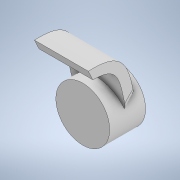
# Autodesk Inventor part: suction_extension
Saved by Autodesk Inventor 2021 (Build 250183000, 183)
## iProperties
Created: 2023-03-20
Part Number: suction_extension
Material: Generic
Document SubType Name: Modeling
Designer: mahmo
Density: 1 g/cm^3
Appearance: Default
Author: mahmo
Autodesk Inventor part; units mm, degrees
ref_plane "YZ Plane" through (0, 0, 0) normal (1, 0, 0) x (0, 1, 0)
ref_plane "XZ Plane" through (0, 0, 0) normal (0, 1, 0) x (-1, 0, 0)
ref_plane "XY Plane" through (0, 0, 0) normal (0, 0, 1) x (1, 0, 0)
sketch "Sketch1" plane through (0, 0, 0) normal (0, 0, 1) x (1, 0, 0)
  circle A0 centre (0, 0) radius 7.5
  dimension "d0" = 15
  constraints: 1 centre point, 1 coincident
  measures "d0" diameter of A0
extrude "Extrusion1" add sketch "Sketch1" along normal blind 10
sketch "Sketch2" plane through (0, 0, 10) normal (0, 0, 1) x (1, 0, 0)
  line L0 (0, 0) -> (0, 15)
  line L1 (-7.5, 16.5) -> (7.5, 16.5)
  line L2 (7.5, 16.5) -> (7.5, 13.5)
  line L3 (7.5, 13.5) -> (-7.5, 13.5)
  line L4 (-7.5, 13.5) -> (-7.5, 16.5)
  line L5 (-7.5, 16.5) -> (7.5, 13.5) construction
  line L6 (7.5, 16.5) -> (-7.5, 13.5) construction
  dimension "d3" = 15
  dimension "d4" = 15
  dimension "d5" = 3
  constraints: 14 end point, 2 midpoint, 2 parallel, 1 horizontal, 1 perpendicular, 1 vertical
  measures "d3" distance of L0.start L0.end
  measures "d4" distance of L2.end L3.end
  measures "d5" distance of L1.end L2.end
sketch "Sketch3" plane through (0, 0, 0) normal (1, 0, 0) x (0, 1, 0)
  line L0 (14.9444, 14.9575) -> (14.9444, 8.9521) construction
  line L1 (14.9444, 8.9521) -> (13.2139, 6.7241) construction
  line L2 (13.2139, 6.7241) -> (8.3998, 6.1566) construction
  line L3 (8.3998, 6.1566) -> (2.9254, 4.977) construction
  spline S0 degree 4 poles (14.9444, 14.9575) (14.9444, 8.9521) (13.2139, 6.7241) (8.3998, 6.1566) (2.9254, 4.977) knots 1 1 1 1 1 2 2 2 2 2
  point P0 (0, 0)
  constraints: 1 vertical, 3 other
sweep "Sweep1" add profiles "Sketch2" path "Sketch3"
fillet "Fillet1" radius 2 2 edges at (7.5, 3.456, 4.2769) (-7.5, 3.456, 4.2769)
body "Solid1"
